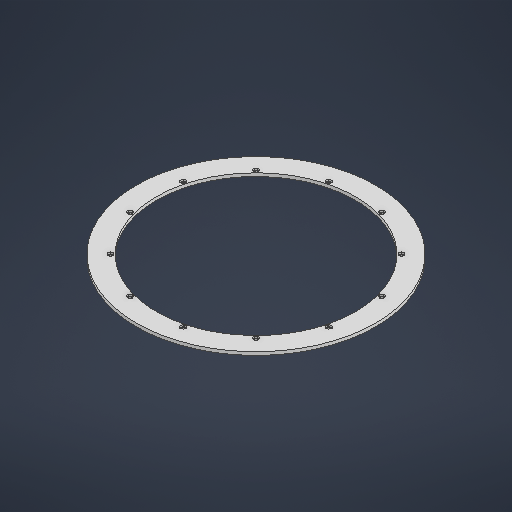
# Autodesk Inventor part: ArmLoopInnerRing
Saved by Autodesk Inventor 2026.1 (Build 301233020, 233B)
## iProperties
Created: 2025-10-20
Part Number: ArmLoopInnerRing
Material: Generic
Document SubType Name: Modeling
Designer: skybound
Density: 1 g/cm^3
Appearance: Default
Author: skybound
Autodesk Inventor part; units mm, degrees
ref_plane "YZ Plane" through (0, 0, 0) normal (1, 0, 0) x (0, 1, 0)
ref_plane "XZ Plane" through (0, 0, 0) normal (0, 1, 0) x (-1, 0, 0)
ref_plane "XY Plane" through (0, 0, 0) normal (0, 0, 1) x (1, 0, 0)
sketch "Sketch1" plane through (0, 0, 0) normal (0, 1, 0) x (-1, 0, 0)
  circle A0 centre (0, 0) radius 150
  circle A1 centre (0, 0) radius 125
  dimension "d0" = 300
  dimension "d1" = 250
  constraints: 2 centre point, 2 coincident
  measures "d0" diameter of A0
  measures "d1" diameter of A1
extrude "Extrusion1" add sketch "Sketch1" along normal blind 4
sketch "Sketch2" plane through (0, 4, 0) normal (0, 1, 0) x (1, 0, 0)
  line L0 (0, 0) -> (124.6044, 33.3877) construction
  line L1 (125.4861, 30.0974) -> (122.1958, 30.979)
  line L2 (122.1958, 30.979) -> (121.3141, 34.2693)
  line L3 (121.3141, 34.2693) -> (123.7228, 36.678)
  line L4 (123.7228, 36.678) -> (127.0131, 35.7963)
  line L5 (127.0131, 35.7963) -> (127.8947, 32.506)
  line L6 (127.8947, 32.506) -> (125.4861, 30.0974)
  line L7 (0, 0) -> (150, 0) construction
  circle A0 centre (0, 0) radius 150 projected
  line L8 (87.9265, 90.3351) -> (88.8081, 93.6254)
  line L9 (90.3351, 87.9265) -> (87.9265, 90.3351)
  line L10 (93.6254, 88.8081) -> (90.3351, 87.9265)
  line L11 (94.5071, 92.0984) -> (93.6254, 88.8081)
  line L12 (92.0984, 94.5071) -> (94.5071, 92.0984)
  line L13 (88.8081, 93.6254) -> (92.0984, 94.5071)
  line L14 (30.979, 122.1958) -> (30.0974, 125.4861)
  line L15 (34.2693, 121.3141) -> (30.979, 122.1958)
  line L16 (36.678, 123.7228) -> (34.2693, 121.3141)
  line L17 (35.7963, 127.0131) -> (36.678, 123.7228)
  line L18 (32.506, 127.8947) -> (35.7963, 127.0131)
  line L19 (30.0974, 125.4861) -> (32.506, 127.8947)
  line L20 (-34.2693, 121.3141) -> (-36.678, 123.7228)
  line L21 (-30.979, 122.1958) -> (-34.2693, 121.3141)
  line L22 (-30.0974, 125.4861) -> (-30.979, 122.1958)
  line L23 (-32.506, 127.8947) -> (-30.0974, 125.4861)
  line L24 (-35.7963, 127.0131) -> (-32.506, 127.8947)
  line L25 (-36.678, 123.7228) -> (-35.7963, 127.0131)
  line L26 (-90.3351, 87.9265) -> (-93.6254, 88.8081)
  line L27 (-87.9265, 90.3351) -> (-90.3351, 87.9265)
  line L28 (-88.8081, 93.6254) -> (-87.9265, 90.3351)
  line L29 (-92.0984, 94.5071) -> (-88.8081, 93.6254)
  line L30 (-94.5071, 92.0984) -> (-92.0984, 94.5071)
  line L31 (-93.6254, 88.8081) -> (-94.5071, 92.0984)
  line L32 (-122.1958, 30.979) -> (-125.4861, 30.0974)
  line L33 (-121.3141, 34.2693) -> (-122.1958, 30.979)
  line L34 (-123.7228, 36.678) -> (-121.3141, 34.2693)
  line L35 (-127.0131, 35.7963) -> (-123.7228, 36.678)
  line L36 (-127.8947, 32.506) -> (-127.0131, 35.7963)
  line L37 (-125.4861, 30.0974) -> (-127.8947, 32.506)
  line L38 (-121.3141, -34.2693) -> (-123.7228, -36.678)
  line L39 (-122.1958, -30.979) -> (-121.3141, -34.2693)
  line L40 (-125.4861, -30.0974) -> (-122.1958, -30.979)
  line L41 (-127.8947, -32.506) -> (-125.4861, -30.0974)
  line L42 (-127.0131, -35.7963) -> (-127.8947, -32.506)
  line L43 (-123.7228, -36.678) -> (-127.0131, -35.7963)
  line L44 (-87.9265, -90.3351) -> (-88.8081, -93.6254)
  line L45 (-90.3351, -87.9265) -> (-87.9265, -90.3351)
  line L46 (-93.6254, -88.8081) -> (-90.3351, -87.9265)
  line L47 (-94.5071, -92.0984) -> (-93.6254, -88.8081)
  line L48 (-92.0984, -94.5071) -> (-94.5071, -92.0984)
  line L49 (-88.8081, -93.6254) -> (-92.0984, -94.5071)
  line L50 (-30.979, -122.1958) -> (-30.0974, -125.4861)
  line L51 (-34.2693, -121.3141) -> (-30.979, -122.1958)
  line L52 (-36.678, -123.7228) -> (-34.2693, -121.3141)
  line L53 (-35.7963, -127.0131) -> (-36.678, -123.7228)
  line L54 (-32.506, -127.8947) -> (-35.7963, -127.0131)
  line L55 (-30.0974, -125.4861) -> (-32.506, -127.8947)
  line L56 (34.2693, -121.3141) -> (36.678, -123.7228)
  line L57 (30.979, -122.1958) -> (34.2693, -121.3141)
  line L58 (30.0974, -125.4861) -> (30.979, -122.1958)
  line L59 (32.506, -127.8947) -> (30.0974, -125.4861)
  line L60 (35.7963, -127.0131) -> (32.506, -127.8947)
  line L61 (36.678, -123.7228) -> (35.7963, -127.0131)
  line L62 (90.3351, -87.9265) -> (93.6254, -88.8081)
  line L63 (87.9265, -90.3351) -> (90.3351, -87.9265)
  line L64 (88.8081, -93.6254) -> (87.9265, -90.3351)
  line L65 (92.0984, -94.5071) -> (88.8081, -93.6254)
  line L66 (94.5071, -92.0984) -> (92.0984, -94.5071)
  line L67 (93.6254, -88.8081) -> (94.5071, -92.0984)
  line L68 (122.1958, -30.979) -> (125.4861, -30.0974)
  line L69 (121.3141, -34.2693) -> (122.1958, -30.979)
  line L70 (123.7228, -36.678) -> (121.3141, -34.2693)
  line L71 (127.0131, -35.7963) -> (123.7228, -36.678)
  line L72 (127.8947, -32.506) -> (127.0131, -35.7963)
  line L73 (125.4861, -30.0974) -> (127.8947, -32.506)
  dimension "d4" = 5.9
  dimension "d5" = 15
  dimension "d6" = 129
  dimension "d9" = 360
  constraints: 148 end point, 1 coincident, 1 horizontal, 1 horizontal alignment, 1 perpendicular, 159 other
  measures "d4" distance between parallel lines of L5 L2
  measures "d5" angle of L7 L0
  measures "d6" distance of L0.start L0.end
extrude "Extrusion2" cut sketch "Sketch2" against normal blind 2 contours L1 L2 L3 L4 L5 L6 | L8 L13 L12 L11 L10 L9 | L14 L19 L18 L17 L16 L15 | L20 L25 L24 L23 L22 L21 | L26 L31 L30 L29 L28 L27 | L32 L37 L36 L35 L34 L33 | L38 L43 L42 L41 L40 L39 | L44 L49 L48 L47 L46 L45 | L50 L55 L54 L53 L52 L51 | L56 L61 L60 L59 L58 L57 | L62 L67 L66 L65 L64 L63 | L68 L73 L72 L71 L70 L69
sketch "Sketch3" plane through (0, 2, 0) normal (0, 1, 0) x (1, 0, 0)
  line L0 (121.3141, 34.2693) -> (123.7228, 36.678) projected
  line L1 (125.4861, 30.0974) -> (122.1958, 30.979) projected
  line L2 (123.7228, 36.678) -> (125.4861, 30.0974) construction
  circle A0 centre (124.6044, 33.3877) radius 1.7
  circle A1 centre (91.2168, 91.2168) radius 1.7
  circle A2 centre (33.3877, 124.6044) radius 1.7
  circle A3 centre (-33.3877, 124.6044) radius 1.7
  circle A4 centre (-91.2168, 91.2168) radius 1.7
  circle A5 centre (-124.6044, 33.3877) radius 1.7
  circle A6 centre (-124.6044, -33.3877) radius 1.7
  circle A7 centre (-91.2168, -91.2168) radius 1.7
  circle A8 centre (-33.3877, -124.6044) radius 1.7
  circle A9 centre (33.3877, -124.6044) radius 1.7
  circle A10 centre (91.2168, -91.2168) radius 1.7
  circle A11 centre (124.6044, -33.3877) radius 1.7
  point P0 (0, 0)
  dimension "d13" = 3.4
  dimension "d16" = 360
  constraints: 12 centre point, 2 end point, 1 midpoint, 25 other
  measures "d13" diameter of A0
extrude "Extrusion3" cut sketch "Sketch3" against normal through all
body "Solid1"
